Autodesk Inventor part; units mm, degrees
(part 3 of 3)
sketch "Skizze2" plane through (0, 0, 1) normal (0, 0, 1) x (1, 0, 0)
  arc A0 (72.421, 47.4152) -> (68.421, 51.4152) centre (68.421, 47.4152) ccw
  line L0 (68.421, 51.4152) -> (-68.421, 51.4152)
  arc A1 (-68.421, 51.4152) -> (-72.421, 47.4152) centre (-68.421, 47.4152) ccw
  line L1 (-72.421, 47.4152) -> (-72.421, -47.4152)
  arc A2 (-72.421, -47.4152) -> (-68.421, -51.4152) centre (-68.421, -47.4152) ccw
  line L2 (-68.421, -51.4152) -> (68.421, -51.4152)
  arc A3 (68.421, -51.4152) -> (72.421, -47.4152) centre (68.421, -47.4152) ccw
  line L3 (72.421, -47.4152) -> (72.421, 47.4152)
  circle A4 centre (68.921, 47.9152) radius 1.5
  circle A5 centre (-68.921, 47.9152) radius 1.4
  circle A6 centre (68.921, -47.9152) radius 1.4
  circle A7 centre (-68.921, -47.9152) radius 1.4
  line L4 (66.921, 45.9152) -> (66.921, -45.9152)
  line L5 (66.921, -45.9152) -> (39.2131, -45.9152)
  arc A8 (38.3736, -45.9152) -> (39.2131, -45.9152) centre (38.7933, -44.5796) ccw
  line L6 (38.3736, -45.9152) -> (20.5131, -45.9152)
  arc A9 (19.6736, -45.9152) -> (20.5131, -45.9152) centre (20.0933, -44.5796) ccw
  line L7 (19.6736, -45.9152) -> (1.8131, -45.9152)
  arc A10 (0.9736, -45.9152) -> (1.8131, -45.9152) centre (1.3933, -44.5796) ccw
  line L8 (0.9736, -45.9152) -> (-16.8869, -45.9152)
  arc A11 (-17.7264, -45.9152) -> (-16.8869, -45.9152) centre (-17.3067, -44.5796) ccw
  line L9 (-17.7264, -45.9152) -> (-35.5869, -45.9152)
  arc A12 (-36.4264, -45.9152) -> (-35.5869, -45.9152) centre (-36.0067, -44.5796) ccw
  line L10 (-36.4264, -45.9152) -> (-54.2869, -45.9152)
  arc A13 (-55.1264, -45.9152) -> (-54.2869, -45.9152) centre (-54.7067, -44.5796) ccw
  line L11 (-55.1264, -45.9152) -> (-66.921, -45.9152)
  line L12 (-66.921, -45.9152) -> (-66.921, 45.9152)
  line L13 (-66.921, 45.9152) -> (66.921, 45.9152)
  point P0 (0, 0)
extrude "Extrusion2" add sketch "Skizze2" along normal blind 5 contours L3 A3 L2 A2 L1 A1 L0 A0 | L4 L5 A8 L6 A9 L7 A10 L8 A11 L9 A12 L10 A13 L11 L12 L13
sketch "Skizze3" plane through (0, 0, 6) normal (0, 0, 1) x (1, 0, 0)
  line L0 (65, 25) -> (15, 25)
  line L1 (15, 25) -> (15, -25)
  line L2 (15, -25) -> (65, -25)
  line L3 (65, -25) -> (65, 25)
  line L4 (65, 25) -> (15, -25) construction
  line L5 (15, 25) -> (65, -25) construction
  point P0 (0, 0)
  point P1 (40, 0)
  dimension "d5" = 50
  dimension "d6" = 50
  dimension "d7" = 40
  constraints: 12 end point, 4 coincident, 2 midpoint, 2 parallel, 1 horizontal, 1 perpendicular
  measures "d5" distance of L2.end L1.end
  measures "d6" distance of L1.end L0.end
  measures "d7" distance of point (0, 0) point (40, 0)
hole "Bohrung1" at (65, 25, 6) at (65, -25, 6) at (15, 25, 6) at (15, -25, 6) direction (0, 0, -1) diameter 4 end through all
sketch "Skizze4" plane through (0, 0, 6) normal (0, 0, 1) x (1, 0, 0)
  circle A0 centre (15, 25) radius 2
  circle A1 centre (65, 25) radius 2
  circle A2 centre (65, -25) radius 2
  line L0 (68.421, 51.4152) -> (-68.421, 51.4152)
  arc A3 (-68.421, 51.4152) -> (-72.421, 47.4152) centre (-68.421, 47.4152) ccw
  line L1 (-72.421, 47.4152) -> (-72.421, -47.4152)
  arc A4 (-72.421, -47.4152) -> (-68.421, -51.4152) centre (-68.421, -47.4152) ccw
  line L2 (-68.421, -51.4152) -> (68.421, -51.4152)
  arc A5 (68.421, -51.4152) -> (72.421, -47.4152) centre (68.421, -47.4152) ccw
  line L3 (72.421, -47.4152) -> (72.421, 47.4152)
  arc A6 (72.421, 47.4152) -> (68.421, 51.4152) centre (68.421, 47.4152) ccw
  circle A7 centre (68.921, 47.9152) radius 1.5
  circle A8 centre (-68.921, 47.9152) radius 1.4
  circle A9 centre (68.921, -47.9152) radius 1.4
  circle A10 centre (-68.921, -47.9152) radius 1.4
  line L4 (67.421, -46.4152) -> (-67.421, -46.4152)
  line L5 (-67.421, -46.4152) -> (-67.421, 46.4152)
  line L6 (-67.421, 46.4152) -> (67.421, 46.4152)
  line L7 (67.421, 46.4152) -> (67.421, -46.4152)
  line L8 (67.421, -46.4152) -> (60.5, -46.4152)
  line L9 (60.5, -46.4152) -> (60.5, 46.4152)
  line L10 (60.5, 46.4152) -> (67.421, 46.4152)
  line L11 (67.421, 46.4152) -> (67.421, -46.4152)
  line L12 (-66.921, 45.9152) -> (66.921, 45.9152)
  line L13 (-67.421, -46.4152) -> (-49.421, -46.4152)
  line L14 (-49.421, -46.4152) -> (-49.421, 45.9152)
  line L15 (-49.421, 45.9152) -> (-67.421, 45.9152)
  line L16 (-67.421, 45.9152) -> (-67.421, -46.4152)
  line L17 (-44.421, 46.4152) -> (10.5, 46.4152)
  line L18 (10.5, 46.4152) -> (10.5, -46.4152)
  line L19 (10.5, -46.4152) -> (-44.421, -46.4152)
  line L20 (-44.421, -46.4152) -> (-44.421, 46.4152)
  line L21 (38.0813, -46.4152) -> (19.5, -46.4152)
  line L22 (19.5, -46.4152) -> (19.5, 46.4152)
  line L23 (19.5, 46.4152) -> (38.0813, 46.4152)
  arc A11 (66.921, 25.5566) -> (66.921, 24.4434) centre (65, 25) ccw
  arc A12 (66.921, -24.4434) -> (66.921, -25.5566) centre (65, -25) ccw
  circle A13 centre (15, 25) radius 2
  circle A14 centre (15, -25) radius 2
  point P0 (0, 0)
  point P1 (-44.421, 45.9152)
  point P2 (10.5, 45.9152)
  point P3 (19.5, 45.9152)
  point P4 (19.5, -46.4152)
  point P5 (60.5, -46.4152)
  point P6 (10.5, 46.4152)
  dimension "d15" = 5
  dimension "d17" = 18
  dimension "d19" = 5
  dimension "d26" = 4.5
  dimension "d27" = 4.5
  dimension "d28" = 4.5
  constraints: 38 end point, 7 parallel, 6 point on line, 4 horizontal, 4 perpendicular, 3 other
  measures "d15" distance between parallel lines of L2 L4
  measures "d17" distance of L15.end L14.end
  measures "d19" distance between parallel lines of L20 L14
  measures "d26" distance from line of L9 A2.centre
  measures "d27" distance from line of A0.centre L22
  measures "d28" distance from line of A0.centre L18
extrude "Extrusion3" cut sketch "Skizze4" against normal through all contours A0 | A1 | A2 | L4 L22 L12 L9 | L12 L22 L6 L9 | L4 L20 L12 L18 | L12 L20 L6 L18 | L4 L14 L12 L20 | L12 L15 L5 L6 L20 | L4 L5 L15 L12 L14
fillet "Rundung1" radius 5 6 edges at (60.5, -46.4152, 3) (10.5, -46.4152, 3) (-67.421, -46.4152, 3) (19.5, -46.4152, 3) (60.5, 46.4152, 3) (-67.421, 46.4152, 3)
